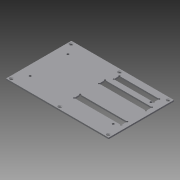
# Autodesk Inventor part: Driver4BusV11Top
Saved by Autodesk Inventor 2013 (Build 170138000, 138)
## iProperties
Created: 2014-07-28
Part Number: Driver4BusV11Top
Material: Generic
Document SubType Name: Sheet Metal
Designer: gsivil
Density: 1 g/cm^3
Sheet Metal Rule: Default
Author: gsivil
Autodesk Inventor part; units mm, degrees
ref_plane "YZ Plane" through (0, 0, 0) normal (1, 0, 0) x (0, 1, 0)
ref_plane "XZ Plane" through (0, 0, 0) normal (0, 1, 0) x (-1, 0, 0)
ref_plane "XY Plane" through (0, 0, 0) normal (0, 0, 1) x (1, 0, 0)
sketch "Sketch1" plane through (0, 0, 0) normal (0, 0, 1) x (1, 0, 0)
  line L0 (93.85, -64.2699) -> (-93.85, -64.2699)
  line L1 (-93.85, -64.2699) -> (-93.85, 55.2301)
  line L2 (-93.85, 55.2301) -> (93.85, 55.2301)
  line L3 (93.85, 55.2301) -> (93.85, -64.2699)
  line L4 (93.85, -64.2699) -> (-93.85, 55.2301) construction
  line L5 (-93.85, -64.2699) -> (93.85, 55.2301) construction
  point P0 (0, 0)
  point P1 (0, -4.5199)
  dimension "d0" = 187.7
  dimension "d1" = 119.5
  constraints: 12 end point, 2 midpoint, 2 parallel, 1 horizontal, 1 perpendicular
  measures "d0" distance of L1.end L2.end
  measures "d1" distance of L0.end L1.end
extrude "Extrusion1" add sketch "Sketch1" along normal mid plane 2.5
hole "Hole2" at (-88.85, -59.3199, 1.25) direction (0, 0, -1) diameter 4 end through all countersink diameter 7 countersink angle 90
hole "Hole3" at (0, -59.2699, 1.25) direction (0, 0, -1) diameter 4 end through all countersink diameter 7 countersink angle 90
hole "Hole4" at (88.9, -59.2699, 1.25) direction (0, 0, -1) diameter 4 end through all countersink diameter 7 countersink angle 90
hole "Hole5" at (-88.9, 50.2301, 1.25) direction (0, 0, -1) diameter 4 end through all countersink diameter 7 countersink angle 90
hole "Hole6" at (0, 50.2301, 1.25) direction (0, 0, -1) diameter 4 end through all countersink diameter 7 countersink angle 90
hole "Hole7" at (88.9, 50.2301, 1.25) direction (0, 0, -1) diameter 4 end through all countersink diameter 7 countersink angle 90
hole "Hole8" at (76.35, -38.2699, 1.25) direction (0, 0, -1) diameter 4 end through all
hole "Hole9" at (76.35, 30.7301, 1.25) direction (0, 0, -1) diameter 4 end through all
hole "Hole10" at (-75.65, -38.2699, 1.25) direction (0, 0, -1) diameter 4 end through all
hole "Hole11" at (-75.65, 30.7301, 1.25) direction (0, 0, -1) diameter 4 end through all
sketch "Sketch5" plane through (0, 0, 1.25) normal (0, 0, 1) x (1, 0, 0)
  circle A0 centre (76.35, -38.2699) radius 2 projected
  line L0 (93.85, -64.2699) -> (93.85, 55.2301) projected
  line L1 (-0.65, -21.7699) -> (85.35, -21.7699)
  line L2 (85.35, -21.7699) -> (85.35, -32.7699)
  line L3 (85.35, -32.7699) -> (-0.65, -32.7699)
  line L4 (-0.65, -32.7699) -> (-0.65, -21.7699)
  point P0 (0, 0)
  dimension "d120" = 8.5
  dimension "d121" = 5.5
  dimension "d122" = 11
  dimension "d123" = 86
  constraints: 8 end point, 2 parallel, 1 horizontal, 1 perpendicular
  measures "d120" distance between parallel lines of L0 L2
  measures "d121" distance from line of A0.centre L3
  measures "d122" distance between parallel lines of L1 L3
  measures "d123" distance between parallel lines of L4 L2
extrude "Cut1" cut sketch "Sketch5" along normal through all both and the other way through all contours L1 L2 L3 L4
pattern_linear "Rectangular Pattern1" count 2 spacing 45.5 along (0, 1, 0) of "Cut1"
sketch "Sketch6" plane through (0, 0, 1.25) normal (0, 0, 1) x (1, 0, 0)
  line L0 (85.35, 23.7301) -> (85.35, 12.7301) projected
  line L1 (85.35, 12.7301) -> (-0.65, 12.7301) projected
  line L2 (5.85, 43.4801) -> (78.85, 43.4801)
  line L3 (78.85, 43.4801) -> (78.85, 33.2301)
  line L4 (78.85, 33.2301) -> (5.85, 33.2301)
  line L5 (5.85, 33.2301) -> (5.85, 43.4801)
  line L6 (-0.65, 23.7301) -> (-0.65, 12.7301) projected
  line L7 (-0.65, 12.7301) -> (85.35, 12.7301) projected
  line L8 (85.35, 12.7301) -> (85.35, 23.7301) projected
  line L9 (85.35, 23.7301) -> (-0.65, 23.7301) projected
  line L10 (-0.65, -21.7699) -> (-0.65, -32.7699) projected
  line L11 (-0.65, -32.7699) -> (85.35, -32.7699) projected
  line L12 (85.35, -32.7699) -> (85.35, -21.7699) projected
  line L13 (85.35, -21.7699) -> (-0.65, -21.7699) projected
  circle A0 centre (-75.65, 30.7301) radius 2 projected
  circle A1 centre (-75.65, -38.2699) radius 2 projected
  circle A2 centre (76.35, 30.7301) radius 2 projected
  circle A3 centre (76.35, -38.2699) radius 2 projected
  line L14 (-93.85, -64.2699) -> (-93.85, 55.2301) projected
  line L15 (-93.85, 55.2301) -> (93.85, 55.2301) projected
  line L16 (93.85, 55.2301) -> (93.85, -64.2699) projected
  line L17 (93.85, -64.2699) -> (-93.85, -64.2699) projected
  circle A4 centre (-88.85, -59.3199) radius 3.5 projected
  circle A5 centre (0, -59.2699) radius 3.5 projected
  circle A6 centre (88.9, -59.2699) radius 3.5 projected
  circle A7 centre (-88.9, 50.2301) radius 3.5 projected
  circle A8 centre (0, 50.2301) radius 3.5 projected
  circle A9 centre (88.9, 50.2301) radius 3.5 projected
  point P0 (0, 0)
  dimension "d129" = 6.5
  dimension "d130" = 20.5
  dimension "d131" = 73
  dimension "d132" = 10.25
  constraints: 8 end point, 2 parallel, 1 horizontal, 1 perpendicular
  measures "d129" distance between parallel lines of L0 L3
  measures "d130" distance between parallel lines of L1 L4
  measures "d131" distance between parallel lines of L3 L5
  measures "d132" distance between parallel lines of L2 L4
extrude "Cut2" cut sketch "Sketch6" against normal through all contours L2 L3 L4 L5
hole "Hole12" at (5.85, 43.4801, 1.25) direction (0, 0, -1) diameter 3 end through all
hole "Hole13" at (78.85, 43.4801, 1.25) direction (0, 0, -1) diameter 3 end through all
hole "Hole14" at (5.85, 33.2301, 1.25) direction (0, 0, -1) diameter 3 end through all
hole "Hole16" at (78.85, 33.2301, 1.25) direction (0, 0, -1) diameter 3 end through all
hole "Hole17" at (-0.65, 23.7301, 1.25) direction (0, 0, -1) diameter 3 end through all
hole "Hole18" at (-0.65, 12.7301, 1.25) direction (0, 0, -1) diameter 3 end through all
hole "Hole19" at (85.35, 12.7301, 1.25) direction (0, 0, -1) diameter 3 end through all
hole "Hole20" at (85.35, 23.7301, 1.25) direction (0, 0, -1) diameter 3 end through all
hole "Hole21" at (-0.65, -21.7699, 1.25) direction (0, 0, -1) diameter 3 end through all
hole "Hole22" at (-0.65, -32.7699, 1.25) direction (0, 0, -1) diameter 3 end through all
hole "Hole23" at (85.35, -21.7699, 1.25) direction (0, 0, -1) diameter 3 end through all
hole "Hole24" at (85.35, -32.7699, 1.25) direction (0, 0, -1) diameter 3 end through all
equation "\"d124\" = Thickness"
equation "\"d133\" = Thickness"
equation "\"d142\" = Thickness"
equation "\"d151\" = Thickness"
equation "\"d160\" = Thickness"
equation "\"d178\" = Thickness"
equation "\"d187\" = Thickness"
equation "\"d196\" = Thickness"
equation "\"d205\" = Thickness"
equation "\"d214\" = Thickness"
equation "\"d223\" = Thickness"
equation "\"d232\" = Thickness"
equation "\"d241\" = Thickness"
equation "\"d250\" = Thickness"
equation "\"BendRadius\" = Thickness"
equation "\"BendReliefWidth\" = Thickness"
equation "\"BendReliefDepth\" = 0.5 * Thickness"
equation "\"CornerReliefSize\" = 4 * Thickness"
equation "\"MinimumRemnant\" = 2 * Thickness"
equation "\"TransitionRadius\" = BendRadius"
equation "\"JacobiRadiusSize\" = Thickness"
equation "\"GapSize\" = Thickness"
equation "\"Thickness\" = 0.5"
body "Solid1"
